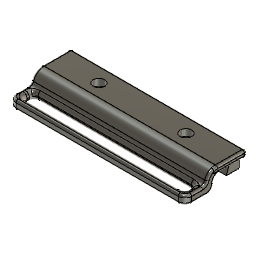
Q.R 2.0 B v2 (Autodesk Fusion 360 design; units mm, degrees)
Autodesk Fusion 360 part; units mm, degrees
sketch "Sketch1" plane through (0, 0, 0) normal (0, 0, 1) x (-1, 0, 0)
  line L0 (-72.0271, 14.75) -> (5.25, 14.75)
  line L1 (6.25, 21.75) -> (-73.0271, 21.75)
  line L2 (-73.0271, 21.75) -> (-73.0271, 8.9009)
  line L3 (-73.0271, 8.9009) -> (6.25, 8.9009)
  line L4 (6.25, 8.9009) -> (6.25, 21.75)
  line L5 (5.25, -0.25) -> (6.25, -0.25)
  line L6 (6.25, 20.75) -> (-13.0359, 20.75)
  arc A0 (-14.4641, 20.75) -> (-13.0359, 20.75) centre (-13.75, 18.25) ccw
  line L7 (-14.4641, 20.75) -> (-52.313, 20.75)
  arc A1 (-53.7413, 20.75) -> (-52.313, 20.75) centre (-53.0271, 18.25) ccw
  line L8 (-73.0271, -0.25) -> (-72.0271, -0.25)
  line L9 (5.25, 14.75) -> (5.25, -0.25)
  line L10 (6.25, -0.25) -> (6.25, 20.75)
  line L11 (-53.7413, 20.75) -> (-73.0271, 20.75)
  line L12 (-73.0271, 20.75) -> (-73.0271, -0.25)
  line L13 (-72.0271, -0.25) -> (-72.0271, 14.75)
  constraint horizontal L1
  constraint vertical L2
  constraint horizontal L3
  constraint vertical L4
extrude "Extrude1" add sketch "Sketch1" along normal blind 2 contours L0 L2 L3 L4 L6 A0 L7 A1 L9 L10 L11 L12 L13 | L0 L3 L9 L13 | L1 L2 L4 L6 A0 L7 A1 L11
sketch "Sketch2" plane through (0, 0, 0) normal (0, 0, -1) x (1, 0, 0)
  line L0 (-6.25, 21.75) -> (-6.25, 8.9009)
  line L1 (-6.25, 8.9009) -> (73.0271, 8.9009)
  line L2 (73.0271, 8.9009) -> (73.0271, 21.75)
  line L3 (73.0271, 21.75) -> (-6.25, 21.75)
  line L4 (-3.2373, 8.9009) -> (69.9912, 8.9009)
  line L5 (69.9912, 8.9009) -> (69.9912, 14.7329)
  line L6 (69.9912, 14.7329) -> (-3.2373, 14.7329)
  line L7 (-3.2373, 14.7329) -> (-3.2373, 8.9009)
  constraint horizontal L4
  constraint vertical L5
  constraint horizontal L6
  constraint vertical L7
  constraint coincident L1 L4.start
extrude "Extrude2" add sketch "Sketch2" along normal blind 6 contours L1 L4 L5 L6 L7
sketch "Sketch3" plane through (69.9912, 0, 0) normal (1, 0, 0) x (0, 1, 0)
  line L0 (-8.9009, 0) -> (-14.7329, 0)
  line L1 (-14.7329, 0) -> (-14.7329, -6)
  line L2 (-14.7329, -6) -> (-8.9009, -6)
  line L3 (-8.9009, -6) -> (-8.9009, 0)
  line L4 (-14.7329, -6) -> (-12.7329, 0)
  dimension "d5" = 2
  constraint coincident L1.end L2.start
  constraint coincident L0 L4.end
  measures "d5" distance of L1 L4.end
extrude "Extrude3" cut sketch "Sketch3" against normal blind 105.5 contours L0 L1 L4
extrude "Extrude4" cut 1 faces at (-3.2373, -12.1223, -4) along direction (1, 0, 0) blind 0.25
extrude "Extrude5" cut 1 faces at (69.9912, -12.1223, -4) along direction (-1, 0, 0) blind 0.25
sketch "Sketch4" plane through (0, -21.75, 0) normal (0, -1, 0) x (1, 0, 0)
  line L0 (-6.25, 0) -> (73.0271, 0)
  line L1 (73.0271, 0) -> (73.0271, 2)
  line L2 (73.0271, 2) -> (-6.25, 2)
  line L3 (-6.25, 2) -> (-6.25, 0)
extrude "Extrude6" add sketch "Sketch4" along normal blind 2
sketch "Sketch5" plane through (0, -23.75, 0) normal (0, -1, 0) x (1, 0, 0)
  line L0 (-6.25, 2) -> (-6.25, 0)
  line L1 (-6.25, 0) -> (73.0271, 0)
  line L2 (73.0271, 0) -> (73.0271, 2)
  line L3 (73.0271, 2) -> (-6.25, 2)
  line L4 (-6.25, 2) -> (73, 2)
  line L5 (73, 2) -> (73, -6)
  line L6 (73, -6) -> (-6.25, -6)
  line L7 (-6.25, -6) -> (-6.25, 2)
  constraint horizontal L4
  constraint vertical L5
  constraint horizontal L6
  constraint vertical L7
  constraint coincident L0.start L3.end
extrude "Extrude7" add sketch "Sketch5" along normal blind 8 contours L0 L1 L3 L4 L5 L7 | L1 L5 L6 L7
sketch "Sketch6" plane through (-6.25, 0, 0) normal (-1, 0, 0) x (0, -1, 0)
  line L0 (8.9009, 0) -> (23.75, 0)
  line L1 (23.75, 0) -> (23.75, -6)
  line L2 (23.75, -6) -> (31.75, -6)
  line L3 (31.75, -6) -> (31.75, 2)
  line L4 (31.75, 2) -> (8.9009, 2)
  line L5 (8.9009, 2) -> (8.9009, 0)
sketch "Sketch7" plane through (0, 0, 2) normal (0, 0, 1) x (-1, 0, 0)
  line L0 (6.25, 8.9009) -> (6.25, 31.75)
  line L1 (6.25, 31.75) -> (-73, 31.75)
  line L2 (-73, 31.75) -> (-73, 23.75)
  line L3 (-73, 23.75) -> (-73.0271, 23.75)
  line L4 (-73.0271, 23.75) -> (-73.0271, 8.9009)
  line L5 (-73.0271, 8.9009) -> (6.25, 8.9009)
  line L6 (6.25, 31.75) -> (-74.9609, 31.75)
  line L7 (-74.9609, 31.75) -> (-74.9609, 26.75)
  line L8 (-74.9609, 26.75) -> (6.25, 26.75)
  line L9 (6.25, 26.75) -> (6.25, 31.75)
  dimension "d16" = 5
  constraint horizontal L6
  constraint vertical L7
  constraint horizontal L8
  constraint vertical L9
  constraint coincident L0.end L1.start
  measures "d16" distance of L0.end L8.end
extrude "Extrude8" cut sketch "Sketch7" against normal blind 4 contours L0 L1 L2 L6 L8 L9
fillet "Fillet1" radius 2 1 edges at (33.375, -26.75, -2)
fillet "Fillet2" radius 3 1 edges at (33.375, -23.75, -6)
fillet "Fillet3" radius 3 1 edges at (33.375, -23.75, 0)
extrude "Extrude9" add 1 faces at (20.1667, -31.75, -4.6667) along direction (0, -1, 0) blind 5
sketch "Sketch8" plane through (0, 0, -2) normal (0, 0, 1) x (-1, 0, 0)
  line L0 (-73, 28.75) -> (6.25, 28.75)
  line L1 (6.25, 28.75) -> (6.25, 36.75)
  line L2 (6.25, 36.75) -> (-73, 36.75)
  line L3 (-73, 36.75) -> (-73, 28.75)
  line L4 (-70, 31.75) -> (3.25, 31.75)
  line L5 (3.25, 31.75) -> (3.25, 33.75)
  line L6 (3.25, 33.75) -> (-70, 33.75)
  line L7 (-70, 33.75) -> (-70, 31.75)
  line L8 (-70, 33.75) -> (-70, 28.75)
  line L9 (3.25, 33.75) -> (3.25, 27)
  dimension "d29" = -3
  constraint coincident L0 L8.end
  constraint perpendicular L0 L8
  constraint perpendicular L0 L9
extrude "Extrude10" cut sketch "Sketch8" against normal blind 18 contours L0 L4 L8 L9 | L4 L5 L6 L7 L8 L9
fillet "Fillet5" radius 2 4 edges at (70, -28.75, -4) (70, -33.75, -4) (-3.25, -28.75, -4) (-3.25, -33.75, -4)
fillet "Fillet6" radius 3 2 edges at (73, -36.75, -4) (-6.25, -36.75, -4)
move_body "Move1" bodies 1 to x (1, 0, 0) y (0, 1, 0) z (0, 0, 1) at (0, -2, 0)
sketch "Sketch11" plane through (0, 0, 0) normal (0, 0, 1) x (-1, 0, 0)
  line L0 (-72.0271, 14.75) -> (5.25, 14.75)
  line L1 (5.25, -0.25) -> (6.25, -0.25)
  line L2 (6.25, 20.75) -> (-13.0359, 20.75)
  arc A0 (-14.4641, 20.75) -> (-13.0359, 20.75) centre (-13.75, 18.25) ccw
  line L3 (-14.4641, 20.75) -> (-52.313, 20.75)
  arc A1 (-53.7413, 20.75) -> (-52.313, 20.75) centre (-53.0271, 18.25) ccw
  line L4 (-73.0271, -0.25) -> (-72.0271, -0.25)
  line L5 (5.25, 14.75) -> (5.25, -0.25)
  line L6 (6.25, -0.25) -> (6.25, 20.75)
  line L7 (-53.7413, 20.75) -> (-73.0271, 20.75)
  line L8 (-73.0271, 20.75) -> (-73.0271, -0.25)
  line L9 (-72.0271, -0.25) -> (-72.0271, 14.75)
sketch "Sketch12" plane through (0, 0, 2) normal (0, 0, 1) x (-1, 0, 0)
  line L0 (6.25, 28.75) -> (-73, 28.75)
  line L1 (-73, 28.75) -> (-73, 25.75)
  line L2 (-73, 25.75) -> (-73.0271, 25.75)
  line L3 (-73.0271, 25.75) -> (-73.0271, 10.9009)
  line L4 (-73.0271, 10.9009) -> (6.25, 10.9009)
  line L5 (6.25, 10.9009) -> (6.25, 28.75)
  circle A0 centre (-53.0271, 18.3009) radius 2.6
  circle A1 centre (-13.75, 18.3009) radius 2.6
  dimension "d38" = 5.2
  dimension "d39" = 5.2
  dimension "d40" = 7.4
  dimension "d41" = 20
  dimension "d42" = 20
  dimension "d43" = 7.4
  measures "d38" diameter of A0
  measures "d39" diameter of A1
  measures "d40" distance of L4 A1.centre
  measures "d41" distance of L5 A1.centre
  measures "d42" distance of L3 A0.centre
  measures "d43" distance of L4 A0.centre
extrude "Extrude11" cut sketch "Sketch12" against normal blind 2 contours A0 | A1
extrude "Extrude12" add 1 faces at (-0.4403, -19.4465, 2) along direction (0, 0, 1) blind 1
fillet "Fillet8" radius 5 1 edges at (33.375, -28.75, 3)
fillet "Fillet9" radius 2 16 edges at (70, -33.25, -2) (69.4142, -35.1642, -2) (33.375, -35.75, -2) (-2.6642, -35.1642, -2) (-3.25, -33.25, -2) (-2.6642, -31.3358, -2) (33.375, -30.75, -2) (69.4142, -31.3358, -2) (-2.6642, -31.3358, -6) (-3.25, -33.25, -6) (-2.6642, -35.1642, -6) (33.375, -35.75, -6) (69.4142, -35.1642, -6) (70, -33.25, -6) (69.4142, -31.3358, -6) (33.375, -30.75, -6)
fillet "Fillet9" radius 1 20 edges at (73, -27.6799, 1.4299) (73, -29.5548, -1.6036) (73, -33.25, -2) (72.1213, -37.8713, -2) (33.375, -38.75, -2) (-5.3713, -37.8713, -2) (-6.25, -33.25, -2) (-6.25, -29.5548, -1.6036) (-6.25, -27.0299, 2.0089) (-6.25, -17.4714, 3) (-6.25, -16.8255, 0) (-6.25, -24.8713, -0.8787) (-6.25, -26.6287, -5.1213) (-6.25, -32.25, -6) (-5.3713, -37.8713, -6) (33.375, -38.75, -6) (72.1213, -37.8713, -6) (73, -32.25, -6) (73, -26.6287, -5.1213) (73, -24.8713, -0.8787)
fillet "Fillet10" radius 1 3 edges at (73.0271, -24.909, 2.9242) (73.0271, -17.4714, 3) (73.0271, -18.3255, 0)
fillet "Fillet11" radius 1 9 edges at (70.8842, -10.9009, 0) (72.7342, -10.9009, 0.2929) (73.0271, -10.9009, 1.5) (72.7342, -10.9009, 2.7071) (33.3886, -10.9009, 3) (-5.9571, -10.9009, 2.7071) (-6.25, -10.9009, 1.5) (-5.9571, -10.9009, 0.2929) (-4.1187, -10.9009, 0)
